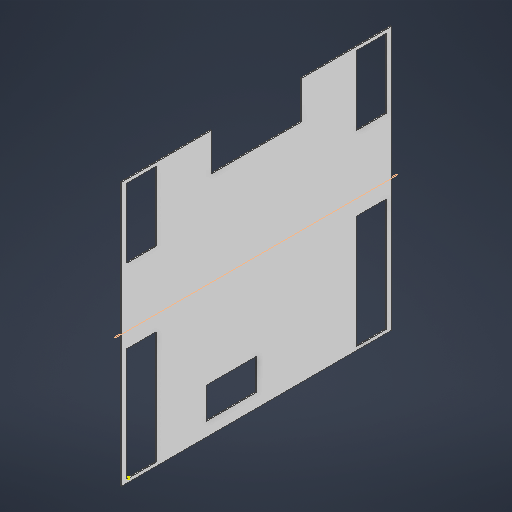
# Autodesk Inventor part: дно 25-26
Saved by Autodesk Inventor 2025 (Build 290162000, 162)
## iProperties
Created: 2025-09-06
Part Number: дно 25-26
Material: Типовые
Document SubType Name: Modeling
Designer: Trene
Density: 1 g/cm^3
Appearance: По умолчанию
Author: Trene
Autodesk Inventor part; units mm, degrees
ref_plane "YZ Plane" through (0, 0, 0) normal (1, 0, 0) x (0, 1, 0)
ref_plane "XZ Plane" through (0, 0, 0) normal (0, 1, 0) x (-1, 0, 0)
ref_plane "XY Plane" through (0, 0, 0) normal (0, 0, 1) x (1, 0, 0)
sketch "Эскиз1" plane through (0, 0, 0) normal (1, 0, 0) x (0, 1, 0)
  line L0 (0, 0) -> (370, 0)
  line L1 (370, 0) -> (370, -370)
  line L2 (370, -370) -> (0, -370)
  line L3 (0, -370) -> (0, 0)
  dimension "d0" = 370
  dimension "d1" = 370
  constraints: 8 end point, 2 parallel, 1 horizontal, 1 perpendicular
  measures "d0" distance of L1.end L2.end
  measures "d1" distance of L0.end L1.end
extrude "Выдавливание1" add sketch "Эскиз1" along normal blind 1.5
sketch "Эскиз3" plane through (1.5, 0, 0) normal (1, 0, 0) x (0, 0, -1)
  line L0 (0, 0) -> (370, 0) projected
  line L1 (8, 0) -> (50, 0)
  line L2 (50, 0) -> (50, 100)
  line L3 (50, 100) -> (8, 100)
  line L4 (8, 100) -> (8, 0)
  line L5 (0, 370) -> (0, 0) projected
  line L6 (370, 370) -> (0, 370) projected
  line L7 (185, 370) -> (185, 0)
  line L8 (0, 185) -> (370, 185)
  line L9 (370, 0) -> (370, 370) projected
  line L10 (362, 0) -> (320, 0)
  line L11 (320, 0) -> (320, 100)
  line L12 (320, 100) -> (362, 100)
  line L13 (362, 100) -> (362, 0)
  line L14 (8, 370) -> (50, 370)
  line L15 (50, 370) -> (50, 270)
  line L16 (50, 270) -> (8, 270)
  line L17 (8, 270) -> (8, 370)
  line L18 (362, 370) -> (320, 370)
  line L19 (320, 370) -> (320, 270)
  line L20 (320, 270) -> (362, 270)
  line L21 (362, 270) -> (362, 370)
  point P0 (362, 370)
  point P1 (8, 370)
  dimension "d9" = 42
  dimension "d10" = 100
  dimension "d13" = 8
  constraints: 36 end point, 12 symmetric about line, 4 midpoint, 2 parallel, 1 horizontal, 1 perpendicular, 1 point on line
  measures "d9" distance of L3.end L2.end
  measures "d10" distance of L2.end L1.end
  measures "d13" distance between parallel lines of L5 L4
extrude "Выдавливание3" cut sketch "Эскиз3" against normal blind 10 contours L4 L3 L2 L0 | L6 L15 L16 L17 | L11 L12 L13 L0 | L6 L21 L20 L19
sketch "Эскиз4" plane through (1.5, 0, 0) normal (1, 0, 0) x (0, 0, -1)
  line L0 (50, 0) -> (320, 0) projected
  line L1 (185, 0) -> (185, 257.6138)
  line L2 (0, 370) -> (0, 0) projected
  line L3 (0, 185) -> (403.9864, 185)
  line L4 (120, 370.5966) -> (250, 370.5966)
  line L5 (250, 370.5966) -> (250, 320.5966)
  line L6 (250, 320.5966) -> (120, 320.5966)
  line L7 (120, 320.5966) -> (120, 370.5966)
  line L8 (120, 370.5966) -> (250, 320.5966) construction
  line L9 (250, 370.5966) -> (120, 320.5966) construction
  point P0 (185, 370)
  point P1 (185, 305.5966)
  dimension "d62" = 50
  dimension "d63" = 130
  constraints: 12 end point, 2 midpoint, 1 horizontal, 1 symmetric about line, 1 vertical, 6 other
  measures "d62" distance between parallel lines of L4 L6
  measures "d63" distance between parallel lines of L7 L5
extrude "Выдавливание4" cut sketch "Эскиз4" against normal blind 10
sketch "Эскиз5" plane through (1.5, 0, 0) normal (1, 0, 0) x (0, 0, -1)
  line L0 (320, 370) -> (250, 370) projected
  line L1 (50, 0) -> (320, 0) projected
  line L2 (185, 0) -> (185, 405.4433)
  line L3 (50, 100) -> (50, 0) projected
  line L4 (320, 100) -> (362, 100) projected
  line L5 (320, 100) -> (362, 100)
  line L6 (362, 100) -> (362, 103)
  line L7 (362, 103) -> (320, 103)
  line L8 (320, 103) -> (320, 100)
  line L9 (50, 100) -> (8, 100)
  line L10 (50, 100) -> (8, 100)
  line L11 (8, 100) -> (8, 103)
  line L12 (8, 103) -> (50, 103)
  line L13 (50, 103) -> (50, 100)
  line L14 (0, 370) -> (0, 0) projected
  line L15 (0, 185) -> (370, 185)
  line L16 (370, 0) -> (370, 370) projected
  line L17 (50, 270) -> (50, 370)
  line L18 (320, 270) -> (362, 270)
  line L19 (320, 270) -> (362, 270)
  line L20 (362, 270) -> (362, 267)
  line L21 (362, 267) -> (320, 267)
  line L22 (320, 267) -> (320, 270)
  line L23 (50, 267) -> (50, 270)
  line L24 (8, 267) -> (50, 267)
  line L25 (50, 270) -> (8, 270)
  line L26 (50, 270) -> (8, 270)
  line L27 (8, 270) -> (8, 267)
  line L28 (320, 0) -> (320, 100) projected
  line L29 (362, 103) -> (320, 103)
  line L30 (320, 103) -> (320, 140)
  line L31 (320, 140) -> (362, 140)
  line L32 (362, 140) -> (362, 103)
  line L33 (8, 103) -> (50, 103)
  line L34 (50, 103) -> (50, 140)
  line L35 (50, 140) -> (8, 140)
  line L36 (8, 140) -> (8, 103)
  point P0 (250, 0)
  point P1 (185, -35.4433)
  dimension "d36" = 42
  dimension "d37" = 3
  constraints: 60 end point, 21 symmetric about line, 4 parallel, 3 midpoint, 2 horizontal, 2 perpendicular, 1 vertical
  measures "d36" distance of L7.end L6.end
  measures "d37" distance of L6.end L5.end
extrude "Выдавливание5" cut sketch "Эскиз5" against normal blind 10 contours L30 L31 L32 L7 | L12 L36 L35 L34
sketch "Эскиз6" plane through (1.5, 0, 0) normal (1, 0, 0) x (0, 0, -1)
  line L0 (320, 370) -> (250, 370) projected
  line L1 (299, 370) -> (259, 370)
  line L2 (259, 370) -> (259, 355)
  line L3 (259, 355) -> (299, 355)
  line L4 (299, 355) -> (299, 370)
  line L5 (250, 320.5966) -> (120, 320.5966) projected
  line L6 (185, 320.5966) -> (185, 152.8583)
  line L7 (71, 370) -> (111, 370)
  line L8 (111, 370) -> (111, 355)
  line L9 (111, 355) -> (71, 355)
  line L10 (71, 355) -> (71, 370)
  line L11 (95.25, 0) -> (95.25, 55) projected
  line L12 (95.25, 0) -> (163.25, 0)
  line L13 (163.25, 0) -> (163.25, 15)
  line L14 (163.25, 15) -> (95.25, 15)
  line L15 (95.25, 15) -> (95.25, 0)
  line L16 (8, 0) -> (50, 0)
  line L17 (50, 0) -> (50, 3)
  line L18 (50, 3) -> (8, 3)
  line L19 (8, 3) -> (8, 0)
  line L20 (362, 0) -> (320, 0)
  line L21 (320, 0) -> (320, 3)
  line L22 (320, 3) -> (362, 3)
  line L23 (362, 3) -> (362, 0)
  line L24 (370, 0) -> (370, 370) projected
  line L25 (370, 0) -> (0, 0)
  line L26 (0, 0) -> (0, -2)
  line L27 (0, -2) -> (370, -2)
  line L28 (370, -2) -> (370, 0)
  line L29 (0, 370) -> (0, 0) projected
  line L30 (0, 185) -> (370, 185)
  line L31 (370, 370) -> (0, 370)
  line L32 (0, 370) -> (0, 372)
  line L33 (0, 372) -> (370, 372)
  line L34 (370, 372) -> (370, 370)
  line L35 (50, 370) -> (50, 367)
  line L36 (50, 367) -> (8, 367)
  line L37 (8, 367) -> (8, 370)
  line L38 (320, 370) -> (320, 367)
  line L39 (320, 367) -> (362, 367)
  line L40 (362, 367) -> (362, 370)
  point P0 (362, 370)
  dimension "d28" = 40
  dimension "d29" = 15
  dimension "d32" = 68
  dimension "d33" = 15
  dimension "d34" = 42
  dimension "d35" = 3
  dimension "d38" = 370
  dimension "d39" = 2
  constraints: 72 end point, 18 symmetric about line, 8 parallel, 4 horizontal, 4 perpendicular, 3 midpoint, 1 vertical
  measures "d28" distance of L3.end L2.end
  measures "d29" distance of L2.end L1.end
  measures "d32" distance of L14.end L13.end
  measures "d33" distance of L13.end L12.end
  measures "d34" distance of L18.end L17.end
  measures "d35" distance of L17.end L16.end
  measures "d38" distance of L27.end L26.end
  measures "d39" distance of L26.end L25.end
extrude "Выдавливание6" add sketch "Эскиз6" against normal up to surface (1.5 mm away) contours L0 L31 L7 L32 L33 L34 | L31 L40 L39 L38 | L4 L3 L2 L0 | L8 L9 L10 L7 | L28 L27 L26 L25 L16 L12 L20 | L20 L21 L22 L23 | L35 L36 L37 L31 | L12 L11 L14 L13 | L19 L18 L17 L16
sketch "Эскиз7" plane through (0, 0, 0) normal (-1, 0, 0) x (0, 0, 1)
  line L0 (0, -2) -> (0, 372) projected
  line L1 (0, 372) -> (-370, 372) projected
  line L2 (-370, -2) -> (-370, 372) projected
  line L3 (-370, -2) -> (0, -2) projected
  line L4 (-362, 3) -> (-362, 100) projected
  line L5 (-320, 100) -> (-320, 3) projected
  line L6 (-320, 3) -> (-362, 3) projected
  line L7 (-320, 367) -> (-320, 270) projected
  line L8 (-362, 270) -> (-362, 367) projected
  line L9 (-362, 367) -> (-320, 367) projected
  line L10 (-250, 370) -> (-120, 370) projected
  line L11 (-120, 370) -> (-120, 320.5966) projected
  line L12 (-120, 320.5966) -> (-250, 320.5966) projected
  line L13 (-250, 320.5966) -> (-250, 370) projected
  line L14 (-8, 3) -> (-50, 3) projected
  line L15 (-50, 3) -> (-50, 100) projected
  line L16 (-8, 100) -> (-8, 3) projected
  line L17 (-50, 367) -> (-8, 367) projected
  line L18 (-8, 367) -> (-8, 270) projected
  line L19 (-50, 270) -> (-50, 367) projected
  line L20 (0, 15) -> (-370, 15)
  line L21 (-362, 100) -> (-320, 100) projected
  line L22 (-320, 270) -> (-362, 270) projected
  line L23 (-50, 100) -> (-8, 100) projected
  line L24 (-8, 270) -> (-50, 270) projected
  point P0 (0, 0)
  point P1 (-8, 15)
  point P2 (-50, 15)
  point P3 (-320, 15)
  point P4 (-362, 15)
  constraints: 2 end point, 2 point on line, 1 perpendicular
extrude "Выдавливание7" cut sketch "Эскиз7" against normal blind 10 contours L3 L2 L20 L4 L6 L5 L15 L14 L16 L0 | L20 L15 L23 L16 | L16 L14 L15 L20 | L20 L5 L6 L4
sketch "Эскиз8" plane through (1.5, 0, 0) normal (1, 0, 0) x (0, 0, -1)
  line L0 (8, 103) -> (8, 140) projected
  line L1 (8, 140) -> (50, 140) projected
  line L2 (50, 140) -> (50, 103) projected
  line L3 (50, 103) -> (8, 103) projected
  line L4 (320, 103) -> (320, 140) projected
  line L5 (320, 140) -> (362, 140) projected
  line L6 (362, 140) -> (362, 103) projected
  line L7 (362, 103) -> (320, 103) projected
  line L8 (8, 367) -> (50, 367) projected
  line L9 (50, 367) -> (50, 270) projected
  line L10 (50, 270) -> (8, 270) projected
  line L11 (8, 270) -> (8, 367) projected
  line L12 (362, 15) -> (370, 15) projected
  line L13 (370, 15) -> (370, 372) projected
  line L14 (370, 372) -> (0, 372) projected
  line L15 (0, 372) -> (0, 15) projected
  line L16 (0, 15) -> (8, 15) projected
  line L17 (8, 15) -> (8, 100) projected
  line L18 (8, 100) -> (50, 100) projected
  line L19 (50, 100) -> (50, 15) projected
  line L20 (50, 15) -> (320, 15) projected
  line L21 (320, 15) -> (320, 100) projected
  line L22 (320, 100) -> (362, 100) projected
  line L23 (362, 100) -> (362, 15) projected
  line L24 (320, 367) -> (362, 367) projected
  line L25 (362, 367) -> (362, 270) projected
  line L26 (362, 270) -> (320, 270) projected
  line L27 (320, 270) -> (320, 367) projected
  line L28 (250, 370) -> (250, 320.5966) projected
  line L29 (250, 320.5966) -> (120, 320.5966) projected
  line L30 (120, 320.5966) -> (120, 370) projected
  line L31 (120, 370) -> (250, 370) projected
  line L32 (362, 100) -> (362, 103)
  line L33 (320, 100) -> (320, 103)
  line L34 (50, 100) -> (50, 103)
  line L35 (8, 100) -> (8, 103)
  line L36 (185, 15) -> (113, 15)
  line L37 (113, 15) -> (113, 60)
  line L38 (113, 60) -> (185, 60)
  line L39 (185, 60) -> (185, 15)
  point P0 (0, 0)
  point P1 (113, 15)
  dimension "d54" = 72
  dimension "d55" = 45
  dimension "d58" = 185
  constraints: 16 end point, 5 parallel, 1 horizontal, 1 midpoint, 1 perpendicular, 1 vertical
  measures "d54" distance of L37.end L38.end
  measures "d55" distance of L36.end L37.end
  measures "d58" distance between parallel lines of L15 L39
extrude "Выдавливание8" cut sketch "Эскиз8" against normal blind 10 contours L3 L34 L18 L35 | L37 L38 L39 L20 | L33 L7 L32 L22
ref_plane "РабПлоскость1" through (1.5, 185, 0) normal (0, 1, 0) x (1, 0, 0)
sketch "Эскиз9" plane through (1.5, 0, 0) normal (1, 0, 0) x (0, 0, -1)
  line L0 (50, 140) -> (50, 15) projected
  line L1 (50, 15) -> (113, 15) projected
  line L2 (113, 15) -> (113, 60) projected
  line L3 (113, 60) -> (185, 60) projected
  line L4 (185, 60) -> (185, 15) projected
  line L5 (185, 15) -> (320, 15) projected
  line L6 (320, 15) -> (320, 140) projected
  line L7 (320, 140) -> (362, 140) projected
  line L8 (362, 140) -> (362, 15) projected
  line L9 (362, 15) -> (370, 15) projected
  line L10 (370, 15) -> (370, 372) projected
  line L11 (370, 372) -> (0, 372) projected
  line L12 (0, 372) -> (0, 15) projected
  line L13 (0, 15) -> (8, 15) projected
  line L14 (8, 15) -> (8, 140) projected
  line L15 (8, 140) -> (50, 140) projected
  line L16 (8, 367) -> (50, 367) projected
  line L17 (50, 367) -> (50, 270) projected
  line L18 (50, 270) -> (8, 270) projected
  line L19 (8, 270) -> (8, 367) projected
  line L20 (320, 367) -> (362, 367) projected
  line L21 (362, 367) -> (362, 270) projected
  line L22 (362, 270) -> (320, 270) projected
  line L23 (320, 270) -> (320, 367) projected
  line L24 (250, 370) -> (250, 320.5966) projected
  line L25 (250, 320.5966) -> (120, 320.5966) projected
  line L26 (120, 320.5966) -> (120, 370) projected
  line L27 (120, 370) -> (250, 370) projected
  line L28 (-74, 185) -> (444, 185) projected
  line L29 (8, 3) -> (50, 3)
  line L30 (50, 3) -> (50, 100)
  line L31 (50, 100) -> (8, 100)
  line L32 (8, 100) -> (8, 3)
  line L33 (320, 3) -> (362, 3)
  line L34 (362, 3) -> (362, 100)
  line L35 (362, 100) -> (320, 100)
  line L36 (320, 100) -> (320, 3)
  line L37 (370, -2) -> (0, -2)
  line L38 (370, -2) -> (370, 15)
  line L39 (0, -2) -> (0, 15)
  line L40 (185, 15) -> (113, 15)
  point P0 (0, 0)
  point P1 (50, 15)
  point P2 (8, 15)
  point P3 (362, 15)
  point P4 (320, 15)
  constraints: 24 end point, 10 symmetric about line, 1 collinear, 1 parallel, 1 vertical
extrude "Выдавливание9" add sketch "Эскиз9" against normal up to surface (1.5 mm away) contours L1 L40 L5 L36 L33 L34 L9 L38 L37 L39 L13 L32 L29 L30
sketch "Эскиз10" plane through (1.5, 0, 0) normal (1, 0, 0) x (0, 0, -1)
  point P0 (0, 0)
sketch "Эскиз11" plane through (1.5, 0, 0) normal (1, 0, 0) x (0, 0, -1)
  line L0 (370, -2) -> (370, 372) projected
  line L1 (370, 372) -> (0, 372) projected
  line L2 (0, 372) -> (0, -2) projected
  line L3 (0, -2) -> (370, -2) projected
  line L4 (113, 15) -> (113, 60) projected
  line L5 (113, 60) -> (185, 60) projected
  line L6 (185, 60) -> (185, 15) projected
  line L7 (185, 15) -> (113, 15) projected
  line L8 (362, 140) -> (362, 3) projected
  line L9 (362, 3) -> (320, 3) projected
  line L10 (320, 3) -> (320, 140) projected
  line L11 (320, 140) -> (362, 140) projected
  line L12 (50, 140) -> (50, 3) projected
  line L13 (50, 3) -> (8, 3) projected
  line L14 (8, 3) -> (8, 140) projected
  line L15 (8, 140) -> (50, 140) projected
  line L16 (8, 367) -> (50, 367) projected
  line L17 (50, 367) -> (50, 270) projected
  line L18 (50, 270) -> (8, 270) projected
  line L19 (8, 270) -> (8, 367) projected
  line L20 (320, 367) -> (362, 367) projected
  line L21 (362, 367) -> (362, 270) projected
  line L22 (362, 270) -> (320, 270) projected
  line L23 (320, 270) -> (320, 367) projected
  line L24 (250, 370) -> (250, 320.5966) projected
  line L25 (250, 320.5966) -> (120, 320.5966) projected
  line L26 (120, 320.5966) -> (120, 370) projected
  line L27 (120, 370) -> (250, 370) projected
  line L28 (320, 140) -> (362, 140)
  line L29 (362, 140) -> (362, 163)
  line L30 (362, 163) -> (320, 163)
  line L31 (320, 163) -> (320, 140)
  line L32 (8, 140) -> (8, 163)
  line L33 (8, 163) -> (50, 163)
  line L34 (50, 163) -> (50, 140)
  line L35 (120, 370) -> (250, 370)
  line L36 (250, 370) -> (250, 392)
  line L37 (250, 392) -> (120, 392)
  line L38 (120, 392) -> (120, 370)
  point P0 (0, 0)
  constraints: 22 end point, 4 parallel, 3 symmetric about line, 2 horizontal, 2 perpendicular
extrude "Выдавливание10" cut sketch "Эскиз11" against normal blind 10 contours L36 L27 L38 L1 | L1 L38 L37 L36 | L11 L31 L30 L29 | L15 L32 L33 L34
sketch "Эскиз12" plane through (1.5, 0, 0) normal (1, 0, 0) x (0, 0, -1)
  line L0 (120, 320.5966) -> (120, 372) projected
  line L1 (120, 372) -> (0, 372) projected
  line L2 (0, 372) -> (0, -2) projected
  line L3 (0, -2) -> (370, -2) projected
  line L4 (370, -2) -> (370, 372) projected
  line L5 (370, 372) -> (250, 372) projected
  line L6 (250, 372) -> (250, 320.5966) projected
  line L7 (250, 320.5966) -> (120, 320.5966) projected
  line L8 (113, 15) -> (113, 60) projected
  line L9 (113, 60) -> (185, 60) projected
  line L10 (185, 60) -> (185, 15) projected
  line L11 (185, 15) -> (113, 15) projected
  line L12 (320, 3) -> (320, 163) projected
  line L13 (320, 163) -> (362, 163) projected
  line L14 (362, 163) -> (362, 3) projected
  line L15 (362, 3) -> (320, 3) projected
  line L16 (8, 3) -> (8, 163) projected
  line L17 (8, 163) -> (50, 163) projected
  line L18 (50, 163) -> (50, 3) projected
  line L19 (50, 3) -> (8, 3) projected
  line L20 (8, 367) -> (50, 367) projected
  line L21 (50, 367) -> (50, 270) projected
  line L22 (50, 270) -> (8, 270) projected
  line L23 (8, 270) -> (8, 367) projected
  line L24 (320, 367) -> (362, 367) projected
  line L25 (362, 367) -> (362, 270) projected
  line L26 (362, 270) -> (320, 270) projected
  line L27 (320, 270) -> (320, 367) projected
  line L28 (0, -2) -> (370, -2)
  line L29 (370, -2) -> (370, -5)
  line L30 (370, -5) -> (0, -5)
  line L31 (0, -5) -> (0, -2)
  line L32 (0, 372) -> (370, 372)
  line L33 (370, 372) -> (370, 375)
  line L34 (370, 375) -> (0, 375)
  line L35 (0, 375) -> (0, 372)
  line L36 (120, 372) -> (250, 372)
  line L37 (250, 372) -> (250, 394)
  line L38 (250, 394) -> (120, 394)
  line L39 (120, 394) -> (120, 372)
  point P0 (0, 0)
  point P1 (120, 375)
  point P2 (250, 375)
  constraints: 24 end point, 6 parallel, 3 horizontal, 3 perpendicular
extrude "Выдавливание11" add sketch "Эскиз12" against normal up to surface (1.5 mm away) contours L1 L35 L34 L39 | L37 L34 L33 L5 | L3 L29 L30 L31
sketch "Эскиз13" plane through (1.5, 0, 0) normal (1, 0, 0) x (0, 0, -1)
  line L0 (120, 320.5966) -> (120, 375) projected
  line L1 (120, 375) -> (0, 375) projected
  line L2 (0, 375) -> (0, -5) projected
  line L3 (0, -5) -> (370, -5) projected
  line L4 (370, -5) -> (370, 375) projected
  line L5 (370, 375) -> (250, 375) projected
  line L6 (250, 375) -> (250, 320.5966) projected
  line L7 (250, 320.5966) -> (120, 320.5966) projected
  line L8 (113, 15) -> (113, 60) projected
  line L9 (113, 60) -> (185, 60) projected
  line L10 (185, 60) -> (185, 15) projected
  line L11 (185, 15) -> (113, 15) projected
  line L12 (320, 3) -> (320, 163) projected
  line L13 (320, 163) -> (362, 163) projected
  line L14 (362, 163) -> (362, 3) projected
  line L15 (362, 3) -> (320, 3) projected
  line L16 (8, 3) -> (8, 163) projected
  line L17 (8, 163) -> (50, 163) projected
  line L18 (50, 163) -> (50, 3) projected
  line L19 (50, 3) -> (8, 3) projected
  line L20 (8, 367) -> (50, 367) projected
  line L21 (50, 367) -> (50, 270) projected
  line L22 (50, 270) -> (8, 270) projected
  line L23 (8, 270) -> (8, 367) projected
  line L24 (320, 367) -> (362, 367) projected
  line L25 (362, 367) -> (362, 270) projected
  line L26 (362, 270) -> (320, 270) projected
  line L27 (320, 270) -> (320, 367) projected
  line L28 (320, 3) -> (362, 3)
  line L29 (362, 3) -> (362, 0)
  line L30 (362, 0) -> (320, 0)
  line L31 (320, 0) -> (320, 3)
  line L32 (8, 3) -> (50, 3)
  line L33 (50, 3) -> (50, 0)
  line L34 (50, 0) -> (8, 0)
  line L35 (8, 0) -> (8, 3)
  line L36 (8, 367) -> (50, 367)
  line L37 (50, 367) -> (50, 370)
  line L38 (50, 370) -> (8, 370)
  line L39 (8, 370) -> (8, 367)
  line L40 (320, 367) -> (362, 367)
  line L41 (362, 367) -> (362, 370)
  line L42 (362, 370) -> (320, 370)
  line L43 (320, 370) -> (320, 367)
  point P0 (0, 0)
  constraints: 32 end point, 8 parallel, 4 horizontal, 4 perpendicular, 2 point on line
extrude "Выдавливание12" cut sketch "Эскиз13" against normal blind 10 contours L15 L29 L30 L31 | L19 L33 L34 L35 | L39 L38 L37 L20 | L43 L42 L41 L24
sketch "Эскиз14" plane through (1.5, 0, 0) normal (1, 0, 0) x (0, 0, -1)
  line L0 (120, 320.5966) -> (120, 375) projected
  line L1 (120, 375) -> (0, 375) projected
  line L2 (0, 375) -> (0, -5) projected
  line L3 (0, -5) -> (370, -5) projected
  line L4 (370, -5) -> (370, 375) projected
  line L5 (370, 375) -> (250, 375) projected
  line L6 (250, 375) -> (250, 320.5966) projected
  line L7 (250, 320.5966) -> (120, 320.5966) projected
  line L8 (113, 15) -> (113, 60) projected
  line L9 (113, 60) -> (185, 60) projected
  line L10 (185, 60) -> (185, 15) projected
  line L11 (185, 15) -> (113, 15) projected
  line L12 (362, 163) -> (362, 0) projected
  line L13 (362, 0) -> (320, 0) projected
  line L14 (320, 0) -> (320, 163) projected
  line L15 (320, 163) -> (362, 163) projected
  line L16 (50, 163) -> (50, 0) projected
  line L17 (50, 0) -> (8, 0) projected
  line L18 (8, 0) -> (8, 163) projected
  line L19 (8, 163) -> (50, 163) projected
  line L20 (8, 270) -> (8, 370) projected
  line L21 (8, 370) -> (50, 370) projected
  line L22 (50, 370) -> (50, 270) projected
  line L23 (50, 270) -> (8, 270) projected
  line L24 (320, 270) -> (320, 370) projected
  line L25 (320, 370) -> (362, 370) projected
  line L26 (362, 370) -> (362, 270) projected
  line L27 (362, 270) -> (320, 270) projected
  line L28 (0, 375) -> (-10, 375)
  line L29 (-10, 375) -> (-10, -5)
  line L30 (-10, -5) -> (0, -5)
  line L31 (0, -5) -> (0, 375)
  line L32 (50, 370) -> (40, 370)
  line L33 (40, 370) -> (40, 0)
  line L34 (40, 0) -> (50, 0)
  line L35 (50, 0) -> (50, 370)
  line L36 (185, 320.5966) -> (185, -45)
  line L37 (370, 375) -> (380, 375)
  line L38 (380, 375) -> (380, -5)
  line L39 (380, -5) -> (370, -5)
  line L40 (330, 370) -> (330, 0)
  point P0 (0, 0)
  point P1 (330, 270)
  point P2 (330, 163)
  point P3 (40, 270)
  point P4 (40, 163)
  constraints: 26 end point, 5 symmetric about line, 4 parallel, 2 horizontal, 2 perpendicular, 1 midpoint, 1 point on line, 1 vertical
extrude "Выдавливание13" add sketch "Эскиз14" against normal up to surface (1.5 mm away) contours L2 L30 L29 L28 | L37 L38 L39 L4 | L40 L13 L14 L15 | L16 L17 L33 L19 | L23 L33 L21 L22 | L24 L25 L40 L27
sketch "Эскиз15" plane through (1.5, 0, 0) normal (1, 0, 0) x (0, 0, -1)
  line L0 (8, 370) -> (8, 270) projected
  line L1 (8, 370) -> (-2, 370)
  line L2 (-2, 370) -> (-2, 270)
  line L3 (-2, 270) -> (8, 270)
  line L4 (8, 270) -> (8, 370)
  line L5 (120, 320.5966) -> (120, 375) projected
  line L6 (120, 375) -> (-10, 375) projected
  line L7 (-10, 375) -> (-10, -5) projected
  line L8 (-10, -5) -> (380, -5) projected
  line L9 (380, -5) -> (380, 375) projected
  line L10 (380, 375) -> (250, 375) projected
  line L11 (250, 375) -> (250, 320.5966) projected
  line L12 (250, 320.5966) -> (120, 320.5966) projected
  line L13 (113, 15) -> (113, 60) projected
  line L14 (113, 60) -> (185, 60) projected
  line L15 (185, 60) -> (185, 15) projected
  line L16 (185, 15) -> (113, 15) projected
  line L17 (362, 163) -> (362, 0) projected
  line L18 (362, 0) -> (330, 0) projected
  line L19 (330, 0) -> (330, 163) projected
  line L20 (330, 163) -> (362, 163) projected
  line L21 (40, 163) -> (40, 0) projected
  line L22 (40, 0) -> (8, 0) projected
  line L23 (8, 0) -> (8, 163) projected
  line L24 (8, 163) -> (40, 163) projected
  line L25 (8, 270) -> (8, 370) projected
  line L26 (8, 370) -> (40, 370) projected
  line L27 (40, 370) -> (40, 270) projected
  line L28 (40, 270) -> (8, 270) projected
  line L29 (330, 370) -> (362, 370) projected
  line L30 (362, 370) -> (362, 270) projected
  line L31 (362, 270) -> (330, 270) projected
  line L32 (330, 270) -> (330, 370) projected
  line L33 (8, 163) -> (-2, 163)
  line L34 (-2, 163) -> (-2, 0)
  line L35 (-2, 0) -> (8, 0)
  line L36 (8, 0) -> (8, 163)
  line L37 (185, 320.5966) -> (185, -34)
  line L38 (362, 370) -> (372, 370)
  line L39 (372, 370) -> (372, 270)
  line L40 (372, 270) -> (362, 270)
  line L41 (362, 163) -> (372, 163)
  line L42 (372, 163) -> (372, 0)
  line L43 (372, 0) -> (362, 0)
  point P0 (0, 0)
  constraints: 30 end point, 7 symmetric about line, 4 parallel, 2 horizontal, 2 perpendicular, 1 midpoint, 1 vertical
extrude "Выдавливание14" cut sketch "Эскиз15" against normal blind 10 contours L0 L3 L2 L1 | L41 L42 L43 L17 | L23 L35 L34 L33 | L38 L39 L40 L30
